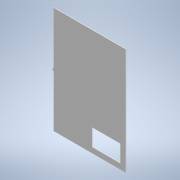
# Autodesk Inventor part: capot
Saved by Autodesk Inventor 2022 (Build 260153000, 153)
## iProperties
Created: 2022-08-02
Part Number: capot
Material: Generic
Document SubType Name: Modeling
Designer: thoma
Density: 1 g/cm^3
Appearance: Default
Author: thoma
Autodesk Inventor part; units mm, degrees
ref_plane "YZ Plane" through (0, 0, 0) normal (1, 0, 0) x (0, 1, 0)
ref_plane "XZ Plane" through (0, 0, 0) normal (0, 1, 0) x (-1, 0, 0)
ref_plane "XY Plane" through (0, 0, 0) normal (0, 0, 1) x (1, 0, 0)
sketch "Sketch1" plane through (0, 0, 0) normal (0, 0, 1) x (1, 0, 0)
  line L0 (0, 0) -> (-672.6812, 0)
  line L1 (-672.6812, 0) -> (-672.6812, -1000)
  line L2 (-672.6812, -1000) -> (0, -1000)
  line L3 (0, -1000) -> (0, 0)
  constraints: 8 end point, 2 parallel, 2 point on line, 1 horizontal, 1 perpendicular, 1 other
extrude "Extrusion1" add sketch "Sketch1" along normal blind 6
sketch "Sketch2" plane through (0, 0, 6) normal (0, 0, 1) x (1, 0, 0)
  line L0 (-50, -800) -> (-305, -800)
  line L1 (-305, -800) -> (-305, -950)
  line L2 (-305, -950) -> (-50, -950)
  line L3 (-50, -950) -> (-50, -800)
  line L4 (-672.6812, -1000) -> (0, -1000) projected
  point P0 (0, 0)
  dimension "d2" = 150
  dimension "d3" = 255
  dimension "d4" = 50
  dimension "d5" = 50
  constraints: 8 end point, 2 parallel, 1 horizontal, 1 perpendicular
  measures "d2" distance of L2.end L0.start
  measures "d3" distance of L0.start L0.end
  measures "d4" distance from line of point (0, 0) L3
  measures "d5" distance between parallel lines of L4 L2
extrude "Extrusion2" cut sketch "Sketch2" against normal through all
body "Solid1"
